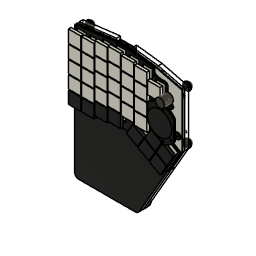
ergothwack-right (requires mirroring) (Autodesk Fusion 360 design; units mm, degrees)
Autodesk Fusion 360 part; units mm, degrees
(part 1 of 6)
sketch "Sketch1" plane through (0, 0, 0) normal (0, 1, 0) x (1, 0, 0)
  line L0 (0, 0) -> (-152.53, 0)
  line L1 (66.3928, -85.1606) -> (66.3928, -83.4672)
  line L2 (66.3928, -83.4672) -> (64.6994, -83.4672)
  line L3 (64.6994, -83.4672) -> (64.6994, -85.1606)
  line L4 (64.6994, -85.1606) -> (66.3928, -85.1606)
  circle A0 centre (65.5461, -86.8539) radius 0.8467
  circle A1 centre (65.5461, -89.3939) radius 0.8467
  circle A2 centre (65.5461, -91.9339) radius 0.8467
  circle A3 centre (65.5461, -94.4739) radius 0.8467
  circle A4 centre (65.5461, -97.0139) radius 0.8467
  circle A5 centre (65.5461, -99.5539) radius 0.8467
  circle A6 centre (65.5461, -102.0939) radius 0.8467
  circle A7 centre (65.5461, -104.6339) radius 0.8467
  circle A8 centre (65.5461, -107.1739) radius 0.8467
  circle A9 centre (65.5461, -109.7139) radius 0.8467
  circle A10 centre (65.5461, -112.2539) radius 0.8467
  line L5 (84.5961, -110.1725) -> (83.3967, -111.3719)
  line L6 (83.3967, -111.3719) -> (84.5961, -112.5714)
  line L7 (84.5961, -112.5714) -> (85.7956, -111.3719)
  line L8 (85.7956, -111.3719) -> (84.5961, -110.1725)
  circle A11 centre (84.5961, -108.8672) radius 0.8467
  circle A12 centre (84.5961, -106.3272) radius 0.8467
  ellipse E0 centre (84.5673, -103.7779) end of major axis (84.5955, -104.6241) minor radius 0.8466
  circle A13 centre (84.5961, -101.2472) radius 0.8467
  circle A14 centre (84.5961, -98.7072) radius 0.8467
  circle A15 centre (84.5961, -96.1672) radius 0.8467
  circle A16 centre (84.5961, -93.6272) radius 0.8467
  circle A17 centre (84.5961, -91.0872) radius 0.8467
  circle A18 centre (84.5961, -88.5472) radius 0.8467
  circle A19 centre (84.5961, -86.0072) radius 0.8467
  circle A20 centre (84.5961, -83.4672) radius 0.8467
  circle A21 centre (83.5378, -112.2539) radius 0.8819
  circle A22 centre (83.5378, -109.7139) radius 0.8819
  circle A23 centre (83.5378, -107.1739) radius 0.8819
  circle A24 centre (83.5378, -104.6339) radius 0.8819
  circle A25 centre (83.5378, -102.0939) radius 0.8819
  circle A26 centre (83.5378, -99.5539) radius 0.8819
  circle A27 centre (83.5378, -97.0139) radius 0.8819
  circle A28 centre (83.5378, -94.4739) radius 0.8819
  circle A29 centre (83.5378, -91.9339) radius 0.8819
  circle A30 centre (83.5378, -89.3939) radius 0.8819
  circle A31 centre (83.5378, -86.8539) radius 0.8819
  circle A32 centre (83.5378, -84.3139) radius 0.8819
  circle A33 centre (68.2978, -84.3139) radius 0.8819
  circle A34 centre (68.2978, -86.8539) radius 0.8819
  circle A35 centre (68.2978, -89.3939) radius 0.8819
  circle A36 centre (68.2978, -91.9339) radius 0.8819
  circle A37 centre (68.2978, -94.4739) radius 0.8819
  circle A38 centre (68.2978, -97.0139) radius 0.8819
  circle A39 centre (68.2978, -99.5539) radius 0.8819
  circle A40 centre (68.2978, -102.0939) radius 0.8819
  circle A41 centre (68.2978, -104.6339) radius 0.8819
  circle A42 centre (68.2978, -107.1739) radius 0.8819
  circle A43 centre (68.2978, -109.7139) radius 0.8819
  circle A44 centre (68.2978, -112.2539) radius 0.8819
  circle A45 centre (80.9978, -89.3939) radius 0.8819
  circle A46 centre (78.4578, -89.3939) radius 0.8819
  circle A47 centre (75.9178, -89.3939) radius 0.8819
  line L9 (86.36, -114.0531) -> (77.3994, -114.0531)
  line L10 (86.36, -81.6328) -> (86.36, -114.0531)
  line L11 (77.3994, -81.6328) -> (86.36, -81.6328)
  line L12 (63.7469, -81.6328) -> (72.7075, -81.6328)
  line L13 (63.7469, -114.0531) -> (63.7469, -81.6681)
  line L14 (72.7075, -114.0531) -> (63.7469, -114.0531)
  circle A48 centre (161.925, -101.6353) radius 0.2469
  circle A49 centre (161.925, -100.8239) radius 0.2469
  circle A50 centre (161.925, -100.0125) radius 0.2469
  circle A51 centre (146.7556, -37.8883) radius 1.5875
  circle A52 centre (115.7464, -33.7256) radius 1.0936
  circle A53 centre (66.4281, -78.105) radius 1.0936
  circle A54 centre (18.8031, -34.0783) radius 1.5875
  circle A55 centre (130.8806, -10.2658) radius 1.5875
  circle A56 centre (123.5781, -102.5878) radius 1.5875
  circle A57 centre (157.6917, -44.4147) radius 1.5875
  circle A58 centre (71.0494, -18.8031) radius 1.0936
  circle A59 centre (95.25, -34.2547) radius 1.0936
  circle A60 centre (146.7556, -76.7997) radius 1.5875
  circle A61 centre (28.3281, -91.2283) radius 1.5875
  circle A62 centre (155.5044, -33.8314) radius 0.8114
  circle A63 centre (155.5044, -36.3714) radius 0.8114
  line L15 (156.3158, -38.5233) -> (156.2806, -38.3822)
  line L16 (156.2806, -38.3822) -> (156.21, -38.2764)
  line L17 (156.21, -38.2764) -> (156.1042, -38.1706)
  line L18 (156.1042, -38.1706) -> (155.9983, -38.1)
  line L19 (155.9983, -38.1) -> (155.8572, -38.0647)
  line L20 (155.8572, -38.0647) -> (155.0458, -38.0647)
  line L21 (155.0458, -38.0647) -> (154.9047, -38.1)
  line L22 (154.9047, -38.1) -> (154.7989, -38.1706)
  line L23 (154.7989, -38.1706) -> (154.6931, -38.2764)
  line L24 (154.6931, -38.2764) -> (154.6225, -38.3822)
  line L25 (154.6225, -38.3822) -> (154.5872, -38.5233)
  line L26 (154.5872, -38.5233) -> (154.5872, -39.3347)
  line L27 (154.5872, -39.3347) -> (154.6225, -39.4758)
  line L28 (154.6225, -39.4758) -> (154.6931, -39.5817)
  line L29 (154.6931, -39.5817) -> (154.7989, -39.6875)
  line L30 (154.7989, -39.6875) -> (154.9047, -39.7581)
  line L31 (154.9047, -39.7581) -> (155.0458, -39.7933)
  line L32 (155.0458, -39.7933) -> (155.8572, -39.7933)
  line L33 (155.8572, -39.7933) -> (155.9983, -39.7581)
  line L34 (155.9983, -39.7581) -> (156.1042, -39.6875)
  line L35 (156.1042, -39.6875) -> (156.21, -39.5817)
  line L36 (156.21, -39.5817) -> (156.2806, -39.4758)
  line L37 (156.2806, -39.4758) -> (156.3158, -39.3347)
  line L38 (156.3158, -39.3347) -> (156.3158, -38.5233)
  circle A64 centre (84.5961, -83.4672) radius 0.8467
  circle A65 centre (84.5961, -86.0072) radius 0.8467
  circle A66 centre (84.5961, -88.5472) radius 0.8467
  circle A67 centre (84.5961, -91.0872) radius 0.8467
  circle A68 centre (84.5961, -93.6272) radius 0.8467
  circle A69 centre (84.5961, -96.1672) radius 0.8467
  circle A70 centre (84.5961, -98.7072) radius 0.8467
  circle A71 centre (84.5961, -101.2472) radius 0.8467
  circle A72 centre (84.5961, -103.7872) radius 0.8467
  circle A73 centre (84.5961, -106.3272) radius 0.8467
  circle A74 centre (84.5961, -108.8672) radius 0.8467
  line L39 (85.4428, -112.2539) -> (85.4428, -110.5253)
  line L40 (85.4428, -110.5253) -> (83.7494, -110.5253)
  line L41 (83.7494, -110.5253) -> (83.7494, -112.2186)
  line L42 (83.7494, -112.2186) -> (85.4428, -112.2186)
  line L43 (85.4428, -112.2186) -> (85.4428, -112.2539)
  circle A75 centre (65.5461, -112.2539) radius 0.8467
  circle A76 centre (65.5461, -109.7139) radius 0.8467
  circle A77 centre (65.5461, -107.1739) radius 0.8467
  circle A78 centre (65.5461, -104.6339) radius 0.8467
  circle A79 centre (65.5461, -102.0939) radius 0.8467
  circle A80 centre (65.5461, -99.5539) radius 0.8467
  circle A81 centre (65.5461, -97.0139) radius 0.8467
  circle A82 centre (65.5461, -94.4739) radius 0.8467
  circle A83 centre (65.5461, -91.9339) radius 0.8467
  circle A84 centre (65.5461, -89.3939) radius 0.8467
  circle A85 centre (65.5461, -86.8539) radius 0.8467
  line L44 (64.6994, -83.4672) -> (64.6994, -85.1606)
  line L45 (64.6994, -85.1606) -> (66.3928, -85.1606)
  line L46 (66.3928, -85.1606) -> (66.3928, -83.4672)
  line L47 (66.3928, -83.4672) -> (64.6994, -83.4672)
  line L48 (130.5278, -107.2444) -> (130.3161, -106.5036)
  line L49 (125.6947, -108.5497) -> (125.483, -107.8089)
  line L50 (160.3728, -84.2433) -> (160.3728, -83.5025)
  line L51 (155.3633, -84.2433) -> (155.3633, -83.5025)
  line L52 (160.3728, -77.7169) -> (160.3728, -76.9761)
  line L53 (155.3633, -77.7169) -> (155.3633, -76.9761)
  circle A86 centre (148.6606, -21.9781) radius 2.6106
  circle A87 centre (139.1356, -5.4681) radius 2.6106
  circle A88 centre (114.3353, -19.7908) radius 2.6106
  circle A89 centre (83.5731, -29.3158) radius 2.6106
  circle A90 centre (56.9031, -29.3158) radius 2.6106
  circle A91 centre (37.8531, -24.5533) radius 2.6106
  circle A92 centre (18.8031, -24.5533) radius 2.6106
  circle A93 centre (132.1506, -31.5383) radius 2.6106
  circle A94 centre (114.0531, -45.9669) radius 2.6106
  circle A95 centre (95.0031, -48.3658) radius 2.6106
  circle A96 centre (75.9531, -50.7294) radius 2.6106
  circle A97 centre (56.9031, -48.3658) radius 2.6106
  circle A98 centre (37.8531, -43.6033) radius 2.6106
  circle A99 centre (18.8031, -43.6033) radius 2.6106
  circle A100 centre (133.1031, -55.4919) radius 2.6106
  circle A101 centre (114.0531, -65.0169) radius 2.6106
  circle A102 centre (95.0031, -67.4158) radius 2.6106
  circle A103 centre (75.9531, -69.7794) radius 2.6106
  circle A104 centre (56.9031, -67.4158) radius 2.6106
  circle A105 centre (37.8531, -62.6533) radius 2.6106
  circle A106 centre (18.8031, -62.6533) radius 2.6106
  circle A107 centre (133.1031, -74.5419) radius 2.6106
  circle A108 centre (114.0531, -84.0669) radius 2.6106
  circle A109 centre (95.0031, -86.4658) radius 2.6106
  circle A110 centre (75.9531, -88.8294) radius 2.6106
  circle A111 centre (56.9031, -86.4658) radius 2.6106
  circle A112 centre (37.8531, -81.7033) radius 2.6106
  circle A113 centre (18.8031, -81.7033) radius 2.6106
  circle A114 centre (133.1031, -93.5919) radius 2.6106
  circle A115 centre (114.0531, -103.1169) radius 2.6106
  circle A116 centre (95.0031, -105.5158) radius 2.6106
  circle A117 centre (75.9531, -107.8794) radius 2.6106
  circle A118 centre (56.9031, -105.5158) radius 2.6106
  circle A119 centre (37.8531, -100.7533) radius 2.6106
  circle A120 centre (18.8031, -100.7533) radius 2.6106
  circle A121 centre (155.5044, -66.5339) radius 0.8114
  circle A122 centre (155.5044, -69.0739) radius 0.8114
  line L54 (156.3158, -71.1906) -> (156.2806, -71.0494)
  line L55 (156.2806, -71.0494) -> (156.21, -70.9436)
  line L56 (156.21, -70.9436) -> (156.1042, -70.8378)
  line L57 (156.1042, -70.8378) -> (155.9983, -70.7672)
  line L58 (155.9983, -70.7672) -> (155.8572, -70.7319)
  line L59 (155.8572, -70.7319) -> (155.0458, -70.7319)
  line L60 (155.0458, -70.7319) -> (154.9047, -70.7672)
  line L61 (154.9047, -70.7672) -> (154.7989, -70.8378)
  line L62 (154.7989, -70.8378) -> (154.6931, -70.9436)
  line L63 (154.6931, -70.9436) -> (154.6225, -71.0494)
  line L64 (154.6225, -71.0494) -> (154.5872, -71.1906)
  line L65 (154.5872, -71.1906) -> (154.5872, -72.0019)
  line L66 (154.5872, -72.0019) -> (154.6225, -72.1431)
  line L67 (154.6225, -72.1431) -> (154.6931, -72.2489)
  line L68 (154.6931, -72.2489) -> (154.7989, -72.3547)
  line L69 (154.7989, -72.3547) -> (154.9047, -72.4253)
  line L70 (154.9047, -72.4253) -> (155.0458, -72.4606)
  line L71 (155.0458, -72.4606) -> (155.8572, -72.4606)
  line L72 (155.8572, -72.4606) -> (155.9983, -72.4253)
  line L73 (155.9983, -72.4253) -> (156.1042, -72.3547)
  line L74 (156.1042, -72.3547) -> (156.21, -72.2489)
  line L75 (156.21, -72.2489) -> (156.2806, -72.1431)
  line L76 (156.2806, -72.1431) -> (156.3158, -72.0019)
  line L77 (156.3158, -72.0019) -> (156.3158, -71.1906)
  circle A123 centre (159.2086, -57.9967) radius 0.9878
  circle A124 centre (159.2086, -52.9872) radius 0.9878
  line L78 (150.6008, -60.0781) -> (150.6008, -62.0889)
  line L79 (150.6008, -62.0889) -> (153.8111, -62.0889)
  line L80 (153.8111, -62.0889) -> (153.8111, -60.0781)
  line L81 (153.8111, -60.0781) -> (150.6008, -60.0781)
  line L82 (150.6008, -48.895) -> (150.6008, -50.9058)
  line L83 (150.6008, -50.9058) -> (153.8111, -50.9058)
  line L84 (153.8111, -50.9058) -> (153.8111, -48.895)
  line L85 (153.8111, -48.895) -> (150.6008, -48.895)
  circle A125 centre (144.7094, -55.4919) radius 0.9878
  circle A126 centre (144.7094, -52.9872) radius 0.9878
  line L86 (143.6864, -57.0089) -> (143.6864, -59.0197)
  line L87 (143.6864, -59.0197) -> (145.6972, -59.0197)
  line L88 (145.6972, -59.0197) -> (145.6972, -57.0089)
  line L89 (145.6972, -57.0089) -> (143.6864, -57.0089)
  circle A127 centre (159.2086, -96.0967) radius 0.9878
  circle A128 centre (159.2086, -91.0872) radius 0.9878
  line L90 (150.6008, -98.1781) -> (150.6008, -100.1889)
  line L91 (150.6008, -100.1889) -> (153.8111, -100.1889)
  line L92 (153.8111, -100.1889) -> (153.8111, -98.1781)
  line L93 (153.8111, -98.1781) -> (150.6008, -98.1781)
  line L94 (150.6008, -86.995) -> (150.6008, -89.0058)
  line L95 (150.6008, -89.0058) -> (153.8111, -89.0058)
  line L96 (153.8111, -89.0058) -> (153.8111, -86.995)
  line L97 (153.8111, -86.995) -> (150.6008, -86.995)
  circle A129 centre (144.7094, -93.5919) radius 0.9878
  circle A130 centre (144.7094, -91.0872) radius 0.9878
  line L98 (143.6864, -95.1089) -> (143.6864, -97.1197)
  line L99 (143.6864, -97.1197) -> (145.6972, -97.1197)
  line L100 (145.6972, -97.1197) -> (145.6972, -95.1089)
  line L101 (145.6972, -95.1089) -> (143.6864, -95.1089)
  circle A131 centre (104.4928, -83.82) radius 0.8467
  line L102 (105.3394, -87.2067) -> (105.3394, -85.5133)
  line L103 (105.3394, -85.5133) -> (103.6461, -85.5133)
  line L104 (103.6461, -85.5133) -> (103.6461, -87.2067)
  line L105 (103.6461, -87.2067) -> (105.3394, -87.2067)
  line L106 (81.4211, -132.3975) -> (92.2514, -132.3975)
  line L107 (92.2514, -132.3975) -> (92.2514, -130.81)
  line L108 (92.2514, -130.81) -> (81.4211, -130.81)
  line L109 (81.4211, -130.81) -> (81.4211, -132.3975)
  line L110 (81.1389, -132.6092) -> (92.5336, -132.6092)
  line L111 (92.5336, -132.6092) -> (92.5336, -130.5983)
  line L112 (92.5336, -130.5983) -> (81.1389, -130.5983)
  line L113 (81.1389, -130.5983) -> (81.1389, -132.6092)
  line L114 (161.7839, -117.9336) -> (161.7839, -131.1628)
  line L115 (9.2428, -117.9336) -> (9.2428, -131.1628)
  line L116 (161.7839, -117.9336) -> (161.7839, -121.92)
  line L117 (9.2428, -117.9336) -> (9.2428, -123.5781)
  line L118 (81.4211, -131.5861) -> (92.2514, -131.5861)
  line L119 (92.2514, -131.5861) -> (92.2514, -129.9986)
  line L120 (92.2514, -129.9986) -> (81.4211, -129.9986)
  line L121 (81.4211, -129.9986) -> (81.4211, -131.5861)
  line L122 (81.1389, -131.7978) -> (92.5336, -131.7978)
  line L123 (92.5336, -131.7978) -> (92.5336, -129.7869)
  line L124 (92.5336, -129.7869) -> (81.1389, -129.7869)
  line L125 (81.1389, -129.7869) -> (81.1389, -131.7978)
  line L126 (80.9978, -130.4925) -> (80.4333, -130.4925)
  line L127 (80.6803, -130.4925) -> (80.6803, -131.4803)
  line L128 (80.6803, -131.4803) -> (80.5744, -131.3392)
  line L129 (80.6097, -131.3392) -> (80.5039, -131.2333)
  line L130 (80.5039, -131.2333) -> (80.3981, -131.1981)
  line L131 (81.8797, -131.4803) -> (81.4211, -131.4803)
  line L132 (81.4211, -131.4803) -> (81.3858, -131.0217)
  line L133 (81.3506, -130.9864) -> (81.3858, -131.0217)
  line L134 (81.4211, -131.0569) -> (81.5269, -131.0922)
  line L135 (81.4917, -131.0922) -> (81.7386, -131.0922)
  line L136 (81.7386, -131.0922) -> (81.8444, -131.0569)
  line L137 (81.8444, -131.0569) -> (81.8797, -131.0217)
  line L138 (81.8797, -130.9864) -> (81.915, -130.8806)
  line L139 (81.9503, -130.9158) -> (81.9503, -130.6689)
  line L140 (81.9503, -130.6689) -> (81.915, -130.5631)
  line L141 (81.8797, -130.5631) -> (81.8444, -130.5278)
  line L142 (81.8444, -130.5278) -> (81.7386, -130.4925)
  line L143 (81.7386, -130.4925) -> (81.4917, -130.4925)
  line L144 (81.4917, -130.4925) -> (81.3858, -130.5278)
  line L145 (81.4211, -130.5278) -> (81.3858, -130.5631)
  line L146 (82.3031, -131.3744) -> (82.3383, -131.4097)
  line L147 (82.3736, -131.445) -> (82.4794, -131.4803)
  line L148 (82.4442, -131.4803) -> (82.6911, -131.4803)
  line L149 (82.6911, -131.4803) -> (82.7969, -131.445)
  line L150 (82.7969, -131.445) -> (82.8322, -131.4097)
  line L151 (82.8322, -131.3744) -> (82.8675, -131.2686)
  line L152 (82.9028, -131.3039) -> (82.9028, -131.1981)
  line L153 (82.9028, -131.1981) -> (82.8675, -131.0569)
  line L154 (82.8322, -131.0569) -> (82.2678, -130.4925)
  line L155 (82.2678, -130.4925) -> (82.9028, -130.4925)
  line L156 (83.3261, -130.5631) -> (83.3614, -130.5278)
  line L157 (83.3614, -130.5278) -> (83.3261, -130.4925)
  line L158 (83.3261, -130.4925) -> (83.2908, -130.5278)
  line L159 (83.2556, -130.5278) -> (83.2908, -130.5631)
  line L160 (83.3261, -130.5631) -> (83.3261, -130.4572)
  line L161 (84.2786, -131.4803) -> (83.82, -131.4803)
  line L162 (83.7847, -131.4803) -> (83.7494, -131.0217)
  line L163 (83.7494, -130.9864) -> (83.7847, -131.0217)
  line L164 (83.7847, -131.0569) -> (83.8906, -131.0922)
  line L165 (83.8906, -131.0922) -> (84.1375, -131.0922)
  line L166 (84.1375, -131.0922) -> (84.2433, -131.0569)
  line L167 (84.2081, -131.0569) -> (84.2433, -131.0217)
  line L168 (84.2786, -130.9864) -> (84.3139, -130.8806)
  line L169 (84.3139, -130.9158) -> (84.3139, -130.6689)
  line L170 (84.3139, -130.6689) -> (84.2786, -130.5631)
  line L171 (84.2786, -130.5631) -> (84.2433, -130.5278)
  line L172 (84.2081, -130.5278) -> (84.1022, -130.4925)
  line L173 (84.1375, -130.4925) -> (83.8906, -130.4925)
  line L174 (83.8906, -130.4925) -> (83.7847, -130.5278)
  line L175 (83.7847, -130.5278) -> (83.7494, -130.5631)
  line L176 (84.6314, -131.4803) -> (85.2664, -131.4803)
  line L177 (85.2664, -131.4803) -> (84.9489, -131.0922)
  line L178 (84.9489, -131.0922) -> (85.09, -131.0922)
  line L179 (85.09, -131.0922) -> (85.1958, -131.0569)
  line L180 (85.1606, -131.0569) -> (85.1958, -131.0217)
  line L181 (85.2311, -130.9864) -> (85.2664, -130.8806)
  line L182 (85.2664, -130.9158) -> (85.2664, -130.6689)
  line L183 (85.2664, -130.6689) -> (85.2311, -130.5631)
  line L184 (85.2311, -130.5631) -> (85.1958, -130.5278)
  line L185 (85.1606, -130.5278) -> (85.0547, -130.4925)
  line L186 (85.09, -130.4925) -> (84.8078, -130.4925)
  line L187 (84.8078, -130.4925) -> (84.7019, -130.5278)
  line L188 (84.7019, -130.5278) -> (84.6667, -130.5631)
  line L189 (85.9014, -131.4803) -> (86.0072, -131.4803)
  line L190 (85.9719, -131.4803) -> (86.0778, -131.445)
  line L191 (86.0778, -131.445) -> (86.1131, -131.4097)
  line L192 (86.1131, -131.3744) -> (86.1483, -131.2686)
  line L193 (86.1836, -131.3039) -> (86.2189, -131.1275)
  line L194 (86.2189, -131.0922) -> (86.2189, -130.8453)
  line L195 (86.2189, -130.8453) -> (86.1836, -130.6689)
  line L196 (86.1836, -130.6689) -> (86.1483, -130.5631)
  line L197 (86.1131, -130.5631) -> (86.0778, -130.5278)
  line L198 (86.0778, -130.5278) -> (85.9719, -130.4925)
  line L199 (85.9719, -130.4925) -> (85.8661, -130.4925)
  line L200 (85.9014, -130.4925) -> (85.7956, -130.5278)
  line L201 (85.7956, -130.5278) -> (85.7603, -130.5631)
  line L202 (85.7603, -130.5631) -> (85.725, -130.6689)
  line L203 (85.6897, -130.6689) -> (85.6544, -130.8453)
  line L204 (85.6544, -130.8453) -> (85.6544, -131.0922)
  line L205 (85.6544, -131.0922) -> (85.6897, -131.2686)
  line L206 (85.6897, -131.3039) -> (85.725, -131.4097)
  line L207 (85.7603, -131.3744) -> (85.7956, -131.4097)
  line L208 (85.7956, -131.445) -> (85.9014, -131.4803)
  line L209 (86.8539, -131.4803) -> (86.9597, -131.4803)
  line L210 (86.9244, -131.4803) -> (87.0303, -131.445)
  line L211 (87.0303, -131.445) -> (87.0656, -131.4097)
  line L212 (87.0656, -131.3744) -> (87.1008, -131.2686)
  line L213 (87.1361, -131.3039) -> (87.1714, -131.1275)
  line L214 (87.1714, -131.0922) -> (87.1714, -130.8453)
  line L215 (87.1714, -130.8453) -> (87.1361, -130.6689)
  line L216 (87.1361, -130.6689) -> (87.1008, -130.5631)
  line L217 (87.0656, -130.5631) -> (87.0303, -130.5278)
  line L218 (87.0303, -130.5278) -> (86.9244, -130.4925)
  line L219 (86.9244, -130.4925) -> (86.8186, -130.4925)
  line L220 (86.8539, -130.4925) -> (86.7481, -130.5278)
  line L221 (86.7481, -130.5278) -> (86.7128, -130.5631)
  line L222 (86.7128, -130.5631) -> (86.6775, -130.6689)
  line L223 (86.6422, -130.6689) -> (86.6069, -130.8453)
  line L224 (86.6069, -130.8453) -> (86.6069, -131.0922)
  line L225 (86.6069, -131.0922) -> (86.6422, -131.2686)
  line L226 (86.6422, -131.3039) -> (86.6775, -131.4097)
  line L227 (86.7128, -131.3744) -> (86.7481, -131.4097)
  line L228 (86.7481, -131.445) -> (86.8539, -131.4803)
  line L229 (88.3708, -130.4925) -> (88.3708, -131.1628)
  line L230 (88.3708, -131.0569) -> (88.4061, -131.0922)
  line L231 (88.4061, -131.0922) -> (88.5119, -131.1275)
  line L232 (88.5119, -131.1275) -> (88.6531, -131.1275)
  line L233 (88.6531, -131.1275) -> (88.7589, -131.0922)
  line L234 (88.7589, -131.0922) -> (88.7942, -130.9864)
  line L235 (88.7942, -130.9864) -> (88.7942, -130.4572)
  line L236 (88.7942, -130.9864) -> (88.8294, -131.0922)
  line L237 (88.8294, -131.0922) -> (88.9353, -131.1275)
  line L238 (88.9353, -131.1275) -> (89.0764, -131.1275)
  line L239 (89.0764, -131.1275) -> (89.1822, -131.0922)
  line L240 (89.1822, -131.0922) -> (89.2175, -130.9864)
  line L241 (89.2175, -130.9864) -> (89.2175, -130.4572)
  line L242 (89.7114, -130.4925) -> (89.7114, -131.1628)
  line L243 (89.7114, -131.0569) -> (89.7467, -131.0922)
  line L244 (89.7467, -131.0922) -> (89.8525, -131.1275)
  line L245 (89.8525, -131.1275) -> (89.9936, -131.1275)
  line L246 (89.9936, -131.1275) -> (90.0994, -131.0922)
  line L247 (90.0642, -131.0922) -> (90.0994, -130.9864)
  line L248 (90.1347, -130.9864) -> (90.1347, -130.4572)
  line L249 (90.1347, -130.9864) -> (90.17, -131.0922)
  line L250 (90.17, -131.0922) -> (90.2758, -131.1275)
  line L251 (90.2758, -131.1275) -> (90.4169, -131.1275)
  line L252 (90.4169, -131.1275) -> (90.5228, -131.0922)
  line L253 (90.4875, -131.0922) -> (90.5228, -130.9864)
  line L254 (90.5581, -130.9864) -> (90.5581, -130.4572)
  line L255 (9.2428, -110.8075) -> (9.2428, -130.3514)
  line L256 (161.7839, -110.8075) -> (161.7839, -130.3514)
  line L257 (9.2428, -129.7869) -> (161.7839, -129.7869)
  line L258 (9.2428, -129.7869) -> (161.7839, -129.7869)
  line L259 (9.2428, -129.7869) -> (10.3717, -130.3867)
  line L260 (9.2428, -129.7869) -> (10.3717, -129.1872)
  line L261 (161.7839, -129.7869) -> (160.655, -129.1872)
  line L262 (161.7839, -129.7869) -> (160.655, -130.3867)
  line L263 (161.7839, -103.1522) -> (161.7839, -110.3136)
  line L264 (-3.474, -61.5853) -> (-3.474, -63.702)
  line L265 (-3.474, -63.702) -> (3.9344, -63.702)
  line L266 (3.9344, -63.702) -> (3.9344, -61.5853)
  line L267 (3.9344, -61.5853) -> (-3.474, -61.5853)
  line L268 (-3.6856, -61.3031) -> (-3.6856, -63.9842)
  line L269 (-3.6856, -63.9842) -> (4.146, -63.9842)
  line L270 (4.146, -63.9842) -> (4.146, -61.3031)
  line L271 (4.146, -61.3031) -> (-3.6856, -61.3031)
  line L272 (0.635, -58.1378) -> (0.635, -58.3142)
  line L273 (0.635, -58.3142) -> (0.5997, -58.42)
  line L274 (0.5997, -58.42) -> (0.5644, -58.4553)
  line L275 (0.5644, -58.4553) -> (0.4233, -58.5611)
  line L276 (0.4233, -58.5611) -> (0.2469, -58.5964)
  line L277 (0.2117, -58.5964) -> (-0.1764, -58.5964)
  line L278 (-0.1764, -58.5964) -> (-0.2822, -58.5611)
  line L279 (-0.2469, -58.5611) -> (-0.2822, -58.5258)
  line L280 (-0.3175, -58.5258) -> (-0.3528, -58.42)
  line L281 (-0.3528, -58.42) -> (-0.3528, -58.2436)
  line L282 (-0.3528, -58.2083) -> (-0.3175, -58.1025)
  line L283 (-0.3175, -58.1378) -> (-0.2822, -58.1025)
  line L284 (-0.2469, -58.0672) -> (-0.1411, -58.0319)
  line L285 (-0.1764, -58.0319) -> (0.0706, -58.0319)
  line L286 (0.0706, -58.0319) -> (0.1764, -58.0672)
  line L287 (0.1764, -58.0672) -> (0.2117, -58.1025)
  line L288 (0.2117, -58.1378) -> (0.2469, -58.2436)
  line L289 (0.2469, -58.2083) -> (0.2469, -58.3847)
  line L290 (0.2469, -58.42) -> (0.2117, -58.5258)
  line L291 (0.2117, -58.5258) -> (0.1764, -58.5611)
  line L292 (0.1764, -58.5611) -> (0.0706, -58.5964)
  line L293 (-0.3528, -59.5136) -> (-0.3528, -59.055)
  line L294 (-0.3528, -59.0197) -> (0.1058, -58.9844)
  line L295 (0.1058, -58.9844) -> (0.0706, -59.0197)
  line L296 (0.0706, -59.0197) -> (0.0353, -59.1256)
  line L297 (0.0353, -59.1256) -> (0.0353, -59.3725)
  line L298 (0.0353, -59.3725) -> (0.0706, -59.4783)
  line L299 (0.0706, -59.4783) -> (0.1058, -59.5136)
  line L300 (0.1058, -59.5136) -> (0.2117, -59.5489)
  line L301 (0.2117, -59.5489) -> (0.4586, -59.5489)
  line L302 (0.4586, -59.5489) -> (0.5644, -59.5136)
  line L303 (0.5644, -59.5136) -> (0.5997, -59.4783)
  line L304 (0.5997, -59.4783) -> (0.635, -59.3725)
  line L305 (0.635, -59.3725) -> (0.635, -59.1256)
  line L306 (0.635, -59.1256) -> (0.5997, -59.0197)
  line L307 (0.5997, -59.0197) -> (0.5644, -58.9844)
  line L308 (0.5644, -59.9722) -> (0.5997, -60.0075)
  line L309 (0.5997, -60.0428) -> (0.635, -60.0075)
  line L310 (0.635, -59.9722) -> (0.5997, -59.9369)
  line L311 (0.5997, -59.9369) -> (0.5644, -59.9722)
  line L312 (0.5644, -59.9722) -> (0.6703, -59.9722)
  line L313 (-0.3528, -60.3603) -> (-0.3528, -60.9953)
  line L314 (-0.3528, -60.9953) -> (0.0353, -60.6778)
  line L315 (0.0353, -60.6425) -> (0.0353, -60.7836)
  line L316 (0.0353, -60.7836) -> (0.0706, -60.8894)
  line L317 (0.0706, -60.8894) -> (0.1058, -60.9247)
  line L318 (0.1058, -60.9247) -> (0.2117, -60.96)
  line L319 (0.2117, -60.9953) -> (0.4586, -60.9953)
  line L320 (0.4586, -60.9953) -> (0.5644, -60.96)
  line L321 (0.5644, -60.9247) -> (0.5997, -60.8894)
  line L322 (0.5997, -60.8894) -> (0.635, -60.7836)
  line L323 (0.635, -60.7836) -> (0.635, -60.5014)
  line L324 (0.635, -60.5014) -> (0.5997, -60.4308)
  line L325 (0.5997, -60.4308) -> (0.5644, -60.3956)
  line L326 (-0.0353, -61.8419) -> (0.635, -61.8419)
  line L327 (-0.3881, -61.595) -> (0.3175, -61.3481)
  line L328 (0.3175, -61.3833) -> (0.3175, -62.0183)
  line L329 (-0.3528, -62.5475) -> (-0.3528, -62.6533)
  line L330 (-0.3528, -62.6533) -> (-0.3175, -62.7592)
  line L331 (-0.3175, -62.7592) -> (-0.2822, -62.7944)
  line L332 (-0.2469, -62.7944) -> (-0.1411, -62.8297)
  line L333 (-0.1764, -62.8297) -> (0, -62.865)
  line L334 (0.0353, -62.9003) -> (0.2822, -62.9003)
  line L335 (0.2469, -62.9003) -> (0.4233, -62.865)
  line L336 (0.4586, -62.8297) -> (0.5644, -62.7944)
  line L337 (0.5644, -62.7944) -> (0.5997, -62.7592)
  line L338 (0.5997, -62.7592) -> (0.635, -62.6533)
  line L339 (0.635, -62.6533) -> (0.635, -62.5475)
  line L340 (0.635, -62.5475) -> (0.5997, -62.4417)
  line L341 (0.5997, -62.4769) -> (0.5644, -62.4417)
  line L342 (0.5644, -62.4064) -> (0.4586, -62.3711)
  line L343 (0.4586, -62.3711) -> (0.2822, -62.3358)
  line L344 (0.2469, -62.3358) -> (0.0353, -62.3358)
  line L345 (0.0353, -62.3358) -> (-0.1411, -62.3711)
  line L346 (-0.1764, -62.3711) -> (-0.2822, -62.4064)
  line L347 (-0.2469, -62.4064) -> (-0.2822, -62.4417)
  line L348 (-0.3175, -62.4769) -> (-0.3528, -62.5475)
  line L349 (-0.3528, -63.5) -> (-0.3528, -63.6058)
  line L350 (-0.3528, -63.6058) -> (-0.3175, -63.7117)
  line L351 (-0.3175, -63.7117) -> (-0.2822, -63.7469)
  line L352 (-0.2469, -63.7469) -> (-0.1411, -63.7822)
  line L353 (-0.1764, -63.7822) -> (0, -63.8175)
  line L354 (0.0353, -63.8528) -> (0.2822, -63.8528)
  line L355 (0.2469, -63.8528) -> (0.4233, -63.8175)
  line L356 (0.4586, -63.7822) -> (0.5644, -63.7469)
  line L357 (0.5644, -63.7469) -> (0.5997, -63.7117)
  line L358 (0.5997, -63.7117) -> (0.635, -63.6058)
  line L359 (0.635, -63.6058) -> (0.635, -63.5)
  line L360 (0.635, -63.5) -> (0.5997, -63.3942)
  line L361 (0.5997, -63.4294) -> (0.5644, -63.3942)
  line L362 (0.5644, -63.3589) -> (0.4586, -63.3236)
  line L363 (0.4586, -63.3236) -> (0.2822, -63.2883)
  line L364 (0.2469, -63.2883) -> (0.0353, -63.2883)
  line L365 (0.0353, -63.2883) -> (-0.1411, -63.3236)
  line L366 (-0.1764, -63.3236) -> (-0.2822, -63.3589)
  line L367 (-0.2469, -63.3589) -> (-0.2822, -63.3942)
  line L368 (-0.3175, -63.4294) -> (-0.3528, -63.5353)
  line L369 (0.635, -65.0169) -> (-0.0353, -65.0169)
  line L370 (0.0706, -65.0169) -> (0.0353, -65.0522)
  line L371 (0.0353, -65.0875) -> (0, -65.1933)
  line L372 (-0.0353, -65.1581) -> (-0.0353, -65.2992)
  line L373 (-0.0353, -65.3344) -> (0, -65.4403)
  line L374 (0.0353, -65.405) -> (0.1411, -65.4403)
  line L375 (0.1058, -65.4756) -> (0.635, -65.4756)
  line L376 (0.1058, -65.4756) -> (0, -65.5108)
  line L377 (0.0353, -65.5108) -> (0, -65.6167)
  line L378 (-0.0353, -65.6167) -> (-0.0353, -65.7578)
  line L379 (-0.0353, -65.7578) -> (0, -65.8636)
  line L380 (0.0353, -65.8283) -> (0.1411, -65.8636)
  line L381 (0.1058, -65.8989) -> (0.635, -65.8989)
  line L382 (0.635, -66.3575) -> (-0.0353, -66.3575)
  line L383 (0.0706, -66.3575) -> (0.0353, -66.4281)
  line L384 (0.0353, -66.4281) -> (0, -66.5339)
  line L385 (-0.0353, -66.4986) -> (-0.0353, -66.6397)
  line L386 (-0.0353, -66.6397) -> (0, -66.7456)
  line L387 (0.0353, -66.7456) -> (0.1411, -66.7808)
  line L388 (0.1058, -66.7808) -> (0.635, -66.7808)
  line L389 (0.1058, -66.7808) -> (0, -66.8161)
  line L390 (0.0353, -66.8514) -> (0, -66.9572)
  line L391 (-0.0353, -66.9219) -> (-0.0353, -67.063)
  line L392 (-0.0353, -67.063) -> (0, -67.1689)
  line L393 (0.0353, -67.1689) -> (0.1411, -67.2042)
  line L394 (0.1058, -67.2394) -> (0.635, -67.2394)
  line L395 (8.7489, -14.9931) -> (0.7408, -14.9931)
  line L396 (8.7489, -110.3136) -> (0.7408, -110.3136)
  line L397 (1.3406, -14.9931) -> (1.3406, -110.3136)
  line L398 (1.3406, -14.9931) -> (1.3406, -110.3136)
  line L399 (1.3406, -14.9931) -> (0.7408, -16.122)
  line L400 (1.3406, -14.9931) -> (1.9403, -16.122)
  line L401 (1.3406, -110.3136) -> (1.9403, -109.1847)
  line L402 (1.3406, -110.3136) -> (0.7408, -109.1847)
  circle A132 centre (66.4281, -78.105) radius 0.9878
  circle A133 centre (115.7464, -33.7256) radius 0.9878
  circle A134 centre (95.25, -34.2547) radius 0.9878
  circle A135 centre (71.0494, -18.8031) radius 0.9878
  circle A136 centre (28.3281, -91.2283) radius 1.5169
  circle A137 centre (18.8031, -34.0783) radius 1.5169
  circle A138 centre (130.9158, -10.2658) radius 1.5169
  circle A139 centre (146.7556, -76.7997) radius 1.5169
  circle A140 centre (157.6917, -44.4147) radius 1.5169
  circle A141 centre (146.7556, -37.8883) radius 1.5169
  circle A142 centre (123.5781, -102.5878) radius 1.5169
  line L403 (9.2428, -105.6569) -> (9.2428, -19.6497)
  line L404 (161.7839, -30.1978) -> (161.7839, -98.4956)
  line L405 (77.8933, -14.9931) -> (103.8578, -14.9931)
  line L406 (9.2428, -14.9931) -> (73.2367, -14.9931)
  line L407 (66.9572, -117.4397) -> (9.2428, -110.3136)
  line L408 (84.9842, -117.4397) -> (66.9572, -117.4397)
  line L409 (123.6133, -112.6772) -> (84.9842, -117.4397)
  line L410 (161.7839, -103.1522) -> (123.6486, -112.6772)
  line L411 (142.6281, 7.5847) -> (103.8578, -14.9931)
  line L412 (161.7839, -25.5411) -> (142.6281, 7.62)
  line L413 (81.4286, 6.2604) -> (95.5897, 6.2604) construction
  line L414 (95.5897, 6.2604) -> (95.5897, 9.7882) construction
  line L415 (95.5897, 9.7882) -> (81.4286, 9.7882) construction
  line L416 (81.4286, 9.7882) -> (81.4286, 6.2604) construction
  line L417 (87.0025, 6.2604) -> (87.0042, 6.2604) construction
  line L418 (87.0042, 6.2604) -> (87.0042, 9.7882) construction
  line L419 (87.0042, 9.7882) -> (87.0025, 9.7882) construction
  line L420 (87.0025, 9.7882) -> (87.0025, 6.2604) construction
  line L421 (90.0364, 6.2604) -> (95.4538, 6.2604) construction
  line L422 (95.4538, 6.2604) -> (95.4538, 9.7882) construction
  line L423 (95.4538, 9.7882) -> (90.0364, 9.7882) construction
  line L424 (90.0364, 9.7882) -> (90.0364, 6.2604) construction
  line L425 (81.1468, 6.4733) -> (95.3079, 6.4733) construction
  line L426 (95.3079, 6.4733) -> (95.3079, 10.0011) construction
  line L427 (95.3079, 10.0011) -> (81.1468, 10.0011) construction
  line L428 (81.1468, 10.0011) -> (81.1468, 6.4733) construction
  line L429 (86.7207, 6.4733) -> (86.7224, 6.4733) construction
  line L430 (86.7224, 6.4733) -> (86.7224, 10.0011) construction
  line L431 (86.7224, 10.0011) -> (86.7207, 10.0011) construction
  line L432 (86.7207, 10.0011) -> (86.7207, 6.4733) construction
  line L433 (90.319, 6.4733) -> (95.7365, 6.4733) construction
  line L434 (95.7365, 6.4733) -> (95.7365, 10.0011) construction
  line L435 (95.7365, 10.0011) -> (90.319, 10.0011) construction
  line L436 (90.319, 10.0011) -> (90.319, 6.4733) construction
  line L437 (81.4286, 5.4429) -> (95.5897, 5.4429) construction
  line L438 (95.5897, 5.4429) -> (95.5897, 8.9706) construction
  line L439 (95.5897, 8.9706) -> (81.4286, 8.9706) construction
  line L440 (81.4286, 8.9706) -> (81.4286, 5.4429) construction
  line L441 (87.0025, 5.4429) -> (87.0042, 5.4429) construction
  line L442 (87.0042, 5.4429) -> (87.0042, 8.9706) construction
  line L443 (87.0042, 8.9706) -> (87.0025, 8.9706) construction
  line L444 (87.0025, 8.9706) -> (87.0025, 5.4429) construction
  line L445 (90.0364, 5.4429) -> (95.4538, 5.4429) construction
  line L446 (95.4538, 5.4429) -> (95.4538, 8.9706) construction
  line L447 (95.4538, 8.9706) -> (90.0364, 8.9706) construction
  line L448 (90.0364, 8.9706) -> (90.0364, 5.4429) construction
  line L449 (81.1468, 5.6558) -> (95.3079, 5.6558) construction
  line L450 (95.3079, 5.6558) -> (95.3079, 9.1836) construction
  line L451 (95.3079, 9.1836) -> (81.1468, 9.1836) construction
  line L452 (81.1468, 9.1836) -> (81.1468, 5.6558) construction
  line L453 (86.7207, 5.6558) -> (86.7224, 5.6558) construction
  line L454 (86.7224, 5.6558) -> (86.7224, 9.1836) construction
  line L455 (86.7224, 9.1836) -> (86.7207, 9.1836) construction
  line L456 (86.7207, 9.1836) -> (86.7207, 5.6558) construction
  line L457 (90.319, 5.6558) -> (95.7365, 5.6558) construction
  line L458 (95.7365, 5.6558) -> (95.7365, 9.1836) construction
  line L459 (95.7365, 9.1836) -> (90.319, 9.1836) construction
  line L460 (90.319, 9.1836) -> (90.319, 5.6558) construction
  line L461 (0.3101, -66.0432) -> (0.3101, -46.8075) construction
  line L462 (0.3101, -46.8075) -> (-3.2177, -46.8075) construction
  line L463 (-3.2177, -46.8075) -> (-3.2177, -66.0432) construction
  line L464 (-3.2177, -66.0432) -> (0.3101, -66.0432) construction
  line L465 (0.0265, -66.2554) -> (0.0265, -53.8186) construction
  line L466 (0.0265, -53.8186) -> (-3.5012, -53.8186) construction
  line L467 (-3.5012, -53.8186) -> (-3.5012, -66.2554) construction
  line L468 (-3.5012, -66.2554) -> (0.0265, -66.2554) construction
  line L469 (4.8596, -66.2554) -> (4.8596, -66.2537) construction
  line L470 (4.8596, -66.2537) -> (1.3318, -66.2537) construction
  line L471 (1.3318, -66.2537) -> (1.3318, -66.2554) construction
  line L472 (1.3318, -66.2554) -> (4.8596, -66.2554) construction
  line L473 (5.6357, -66.2554) -> (5.6357, -60.838) construction
  line L474 (5.6357, -60.838) -> (2.1079, -60.838) construction
  line L475 (2.1079, -60.838) -> (2.1079, -66.2554) construction
  line L476 (2.1079, -66.2554) -> (5.6357, -66.2554) construction
  line L477 (9.2428, -110.3136) -> (9.2428, -14.9931)
  line L478 (9.2428, -14.9931) -> (103.8578, -14.9931)
  line L479 (103.8578, -14.9931) -> (142.6281, 7.5847)
  line L480 (142.6281, 7.5847) -> (161.7839, -25.5411)
  line L481 (161.7839, -25.5411) -> (161.7839, -103.1522)
  line L482 (123.6486, -112.6772) -> (84.9842, -117.4397)
  line L483 (84.9842, -117.4397) -> (66.9572, -117.4397)
  line L484 (9.2428, -110.3136) -> (66.9572, -117.4397)
  line L485 (63.7469, -81.6328) -> (63.5469, -81.6328)
  line L486 (63.5469, -81.6328) -> (63.5469, -81.4328)
  line L487 (63.5469, -81.4328) -> (63.7469, -81.4328)
  line L488 (63.7469, -81.4328) -> (63.7469, -81.6328)
  line L489 (86.36, -81.6328) -> (86.56, -81.6328)
  line L490 (86.56, -81.6328) -> (86.56, -81.4328)
  line L491 (86.56, -81.4328) -> (86.36, -81.4328)
  line L492 (86.36, -81.4328) -> (86.36, -81.6328)
  line L493 (63.5469, -81.6328) -> (63.5469, -117.0186)
  line L494 (63.7469, -81.4328) -> (86.36, -81.4328)
  line L495 (86.56, -81.6328) -> (86.56, -117.2454)
  line L496 (63.5469, -81.4328) -> (57.5469, -81.4328)
  line L497 (57.5469, -81.4328) -> (57.5469, -87.4328)
  line L498 (86.56, -81.4328) -> (92.56, -81.4328)
  line L499 (9.2428, -51.1815) -> (27.2428, -51.1815)
  line L500 (161.7839, -48.2006) -> (143.7839, -48.2006)
  line L501 (57.5469, -81.4328) -> (27.2428, -81.4328)
  line L502 (27.2428, -81.4328) -> (27.2428, -51.1815)
  line L503 (143.7839, -48.2006) -> (143.7839, -81.4328)
  line L504 (143.7839, -81.4328) -> (92.56, -81.4328)
  line L505 (27.2428, -51.1815) -> (27.2428, -15.9328)
  line L506 (27.2428, -15.9328) -> (143.7839, -15.9328)
  line L507 (143.7839, -15.9328) -> (143.7839, -48.2006)
  line L508 (9.2428, -14.9931) -> (9.2428, 80.3275)
  line L509 (142.6281, 7.5847) -> (100.6075, 80.3275)
  line L510 (9.2428, 80.3275) -> (100.6075, 80.3275)
  line L511 (9.2428, 80.3275) -> (15.2428, 80.3275)
  line L512 (15.2428, 80.3275) -> (15.2428, 74.3275)
  line L513 (15.2428, 74.3275) -> (9.2428, 74.3275)
  line L514 (9.2428, 74.3275) -> (9.2428, 80.3275)
  line L515 (97.1443, 80.3275) -> (97.1443, 74.3275)
  line L516 (97.1443, 74.3275) -> (104.0735, 74.3275)
  circle A143 centre (97.1443, 74.3275) radius 6
  circle A144 centre (155.7839, -98.4665) radius 6
  circle A145 centre (15.2428, -105.0089) radius 6
  circle A146 centre (15.2428, 74.3275) radius 6
  circle A147 centre (155.7839, -27.151) radius 6
  line L517 (157.9757, -18.9558) -> (147.6976, -24.893)
  line L518 (161.7839, -33.151) -> (153.5462, -33.151)
  line L519 (161.7839, -92.4665) -> (149.7839, -92.4665)
  line L520 (149.7839, -92.4665) -> (149.7839, -106.1494)
  line L521 (9.2428, -99.0089) -> (21.2428, -99.0089)
  line L522 (21.2428, -99.0089) -> (21.2428, -111.7953)
  line L523 (91.1443, 80.3275) -> (91.1443, 68.3275)
  line L524 (91.1443, 68.3275) -> (107.5394, 68.3275)
  line L525 (9.2428, 68.3275) -> (21.2428, 68.3275)
  line L526 (21.2428, 68.3275) -> (21.2428, 80.3275)
  line L527 (27.2428, -81.4328) -> (21.2428, -81.4328)
  line L528 (21.2428, -81.4328) -> (21.2428, -75.4328)
  line L529 (27.2428, -15.9328) -> (21.2428, -15.9328)
  line L530 (21.2428, -15.9328) -> (21.2428, -21.9328)
  line L531 (143.7839, -15.9328) -> (143.7839, -9.9328)
  line L532 (143.7839, -9.9328) -> (119.7839, -9.9328)
  line L533 (143.7839, -81.4328) -> (86.56, -81.4328)
  line L534 (86.56, -81.4328) -> (86.56, -89.4328)
  line L535 (86.56, -89.4328) -> (143.7839, -89.4328)
  line L536 (143.7839, -89.4328) -> (143.7839, -81.4328)
  circle A148 centre (143.7839, -87.4328) radius 2
  circle A149 centre (88.56, -87.4328) radius 2
  circle A150 centre (141.7839, -15.9328) radius 2
  circle A151 centre (27.2428, -17.9328) radius 2
  circle A152 centre (29.2428, -81.4328) radius 2
  circle A153 centre (21.2428, -75.4328) radius 2.5
  circle A154 centre (21.2428, -21.9328) radius 2.5
  circle A155 centre (119.7839, -9.9328) radius 2.5
  circle A156 centre (57.5469, -87.4328) radius 2.5
  line L537 (92.56, -89.4328) -> (92.56, -95.4328)
  circle A157 centre (92.56, -95.4328) radius 2.5
  line L538 (143.7839, -89.4328) -> (149.7839, -89.4328)
  line L539 (149.7839, -89.4328) -> (149.7839, -83.4328)
  circle A158 centre (149.7839, -83.4328) radius 2.5
  line L540 (143.7839, -89.4328) -> (150.9524, -85.6429)
  line L541 (149.7839, -80.9328) -> (143.7839, -80.9328)
  line L542 (86.56, -89.4328) -> (90.3499, -96.6012)
  line L543 (92.56, -89.4328) -> (98.56, -89.4328)
  line L544 (98.56, -89.4328) -> (94.7701, -96.6012)
  line L545 (63.5469, -81.4328) -> (59.7571, -88.6012)
  line L546 (57.5469, -81.4328) -> (51.5469, -81.4328)
  line L547 (51.5469, -81.4328) -> (55.3368, -88.6012)
  line L548 (27.2428, -81.4328) -> (20.0743, -77.6429)
  line L549 (119.7839, -9.9328) -> (119.7839, -15.9328)
  line L550 (119.7839, -15.9328) -> (125.7839, -15.9328)
  line L551 (119.7839, -15.9328) -> (113.7839, -15.9328)
  line L552 (113.7839, -15.9328) -> (117.5738, -8.7643)
  line L553 (125.7839, -15.9328) -> (121.994, -8.7643)
  line L554 (27.2428, -15.9328) -> (20.0743, -19.7226)
  line L555 (21.2428, -21.9328) -> (27.2428, -21.9328)
  line L556 (27.2428, -21.9328) -> (27.2428, -27.9328)
  line L557 (27.2428, -27.9328) -> (20.0743, -24.1429)
  line L558 (21.2428, -75.4328) -> (27.2428, -75.4328)
  line L559 (27.2428, -75.4328) -> (27.2428, -69.4328)
  line L560 (27.2428, -69.4328) -> (20.0743, -73.2226)
  line L561 (18.8031, -81.7033) -> (9.2428, -81.7033)
  line L562 (142.7339, -107.9103) -> (142.7339, -30.6526)
  line L563 (161.7839, -25.5411) -> (155.7839, -27.151)
  line L564 (155.7839, -27.151) -> (142.7339, -30.6526)
  line L565 (146.7556, -76.7997) -> (142.7339, -76.7997)
  line L566 (146.7556, -76.7997) -> (150.7772, -76.7997)
  line L567 (150.7772, -76.7997) -> (150.7772, -74.7889)
  line L568 (150.7772, -76.7997) -> (150.7772, -78.8106)
  line L569 (142.7339, -82.8322) -> (150.7772, -78.8106)
  line L570 (150.7772, -74.7889) -> (142.7339, -70.7672)
  line L571 (142.7339, -76.7997) -> (142.7339, -70.7672)
  line L572 (142.7339, -107.9103) -> (123.6486, -112.6772)
  line L573 (123.6486, -112.6772) -> (118.0197, -90.1409)
  line L574 (161.7839, -103.1522) -> (145.5587, -103.1522)
  line L575 (126.1031, -100.5919) -> (140.1031, -100.5919)
  line L576 (140.1031, -100.5919) -> (140.1031, -86.5919)
  line L577 (140.1031, -86.5919) -> (126.1031, -86.5919)
  line L578 (126.1031, -86.5919) -> (126.1031, -100.5919)
  line L579 (140.1031, -100.5919) -> (140.1031, -103.2228)
  line L580 (121.9175, -105.7465) -> (132.0216, -103.2228)
  line L581 (132.0216, -103.2228) -> (140.1031, -103.2228)
  line L582 (140.1031, -103.2228) -> (142.7339, -103.2228)
  line L583 (125.5889, -108.1793) -> (124.8013, -105.0262)
  line L584 (146.7556, -37.8883) -> (150.7772, -37.8883)
  line L585 (150.7772, -37.8883) -> (150.7772, -40.3375)
  line L586 (143.7839, -37.8883) -> (143.7839, -43.9208)
  line L587 (146.7556, -37.8883) -> (143.7839, -37.8883)
  line L588 (150.7772, -37.8883) -> (150.7772, -28.4944)
  line L589 (144.7094, -55.4919) -> (144.7094, -48.4919)
  line L590 (144.7094, -48.4919) -> (157.6917, -48.4919)
  line L591 (157.6917, -48.4919) -> (161.7839, -46.6688)
  line L592 (161.7839, -46.6688) -> (161.7839, -42.1606)
  line L593 (150.7772, -40.3375) -> (157.6917, -40.3375)
  line L594 (157.6917, -40.3375) -> (161.7839, -42.1606)
  line L595 (157.6917, -44.4147) -> (157.6917, -48.4919)
  line L596 (157.6917, -44.4147) -> (157.6917, -40.3375)
  line L597 (143.7839, -43.9208) -> (142.7339, -43.9208)
  line L598 (142.7339, -43.9208) -> (150.7772, -40.3375)
  line L599 (144.7094, -48.4919) -> (142.7339, -48.4919)
  line L600 (157.6917, -48.4919) -> (161.7839, -48.4919)
  line L601 (157.6917, -40.3375) -> (161.7839, -40.3375)
  line L602 (146.7556, -76.7997) -> (146.7556, -80.8214)
  line L603 (146.7556, -76.7997) -> (146.7556, -72.7781)
  line L604 (146.7556, -72.7781) -> (142.7339, -72.7781)
  line L605 (146.7556, -72.7781) -> (150.7772, -72.7781)
  line L606 (150.7772, -72.7781) -> (150.7772, -74.7889)
  line L607 (150.7772, -78.8106) -> (150.7772, -80.8214)
  line L608 (150.7772, -80.8214) -> (146.7556, -80.8214)
  line L609 (142.7339, -80.8214) -> (146.7556, -80.8214)
  point P0 (66.3928, -86.8539)
  point P1 (66.3928, -89.3939)
  point P2 (66.3928, -91.9339)
  point P3 (66.3928, -94.4739)
  point P4 (66.3928, -97.0139)
  point P5 (66.3928, -99.5539)
  point P6 (66.3928, -102.0939)
  point P7 (66.3928, -104.6339)
  point P8 (66.3928, -107.1739)
  point P9 (66.3928, -109.7139)
  point P10 (66.3928, -112.2539)
  point P11 (85.4428, -108.8672)
  point P12 (85.4428, -106.3272)
  point P13 (84.5955, -104.6241)
  point P14 (85.4428, -101.2472)
  point P15 (85.4428, -98.7072)
  point P16 (85.4428, -96.1672)
  point P17 (85.4428, -93.6272)
  point P18 (85.4428, -91.0872)
  point P19 (85.4428, -88.5472)
  point P20 (85.4428, -86.0072)
  point P21 (85.4428, -83.4672)
  point P22 (84.4197, -112.2539)
  point P23 (84.4197, -109.7139)
  point P24 (84.4197, -107.1739)
  point P25 (84.4197, -104.6339)
  point P26 (84.4197, -102.0939)
  point P27 (84.4197, -99.5539)
  point P28 (84.4197, -97.0139)
  point P29 (84.4197, -94.4739)
  point P30 (84.4197, -91.9339)
  point P31 (84.4197, -89.3939)
  point P32 (84.4197, -86.8539)
  point P33 (84.4197, -84.3139)
  point P34 (69.1797, -84.3139)
  point P35 (69.1797, -86.8539)
  point P36 (69.1797, -89.3939)
  point P37 (69.1797, -91.9339)
  point P38 (69.1797, -94.4739)
  point P39 (69.1797, -97.0139)
  point P40 (69.1797, -99.5539)
  point P41 (69.1797, -102.0939)
  point P42 (69.1797, -104.6339)
  point P43 (69.1797, -107.1739)
  point P44 (69.1797, -109.7139)
  point P45 (69.1797, -112.2539)
  point P46 (81.8797, -89.3939)
  point P47 (79.3397, -89.3939)
  point P48 (76.7997, -89.3939)
  point P49 (162.1719, -101.6353)
  point P50 (162.1719, -100.8239)
  point P51 (162.1719, -100.0125)
  point P52 (148.3431, -37.8883)
  point P53 (116.84, -33.7256)
  point P54 (67.5217, -78.105)
  point P55 (20.3906, -34.0783)
  point P56 (132.4681, -10.2658)
  point P57 (125.1656, -102.5878)
  point P58 (159.2792, -44.4147)
  point P59 (72.1431, -18.8031)
  point P60 (96.3436, -34.2547)
  point P61 (148.3431, -76.7997)
  point P62 (29.9156, -91.2283)
  point P63 (156.3158, -33.8314)
  point P64 (156.3158, -36.3714)
  point P65 (85.4428, -103.7872)
  point P66 (151.2711, -21.9781)
  point P67 (141.7461, -5.4681)
  point P68 (116.9458, -19.7908)
  point P69 (86.1836, -29.3158)
  point P70 (59.5136, -29.3158)
  point P71 (40.4636, -24.5533)
  point P72 (21.4136, -24.5533)
  point P73 (134.7611, -31.5383)
  point P74 (116.6636, -45.9669)
  point P75 (97.6136, -48.3658)
  point P76 (78.5636, -50.7294)
  point P77 (59.5136, -48.3658)
  point P78 (40.4636, -43.6033)
  point P79 (21.4136, -43.6033)
  point P80 (135.7136, -55.4919)
  point P81 (116.6636, -65.0169)
  point P82 (97.6136, -67.4158)
  point P83 (78.5636, -69.7794)
  point P84 (59.5136, -67.4158)
  point P85 (40.4636, -62.6533)
  point P86 (21.4136, -62.6533)
  point P87 (135.7136, -74.5419)
  point P88 (116.6636, -84.0669)
  point P89 (97.6136, -86.4658)
  point P90 (78.5636, -88.8294)
  point P91 (59.5136, -86.4658)
  point P92 (40.4636, -81.7033)
  point P93 (21.4136, -81.7033)
  point P94 (135.7136, -93.5919)
  point P95 (116.6636, -103.1169)
  point P96 (97.6136, -105.5158)
  point P97 (78.5636, -107.8794)
  point P98 (59.5136, -105.5158)
  point P99 (40.4636, -100.7533)
  point P100 (21.4136, -100.7533)
  point P101 (156.3158, -66.5339)
  point P102 (156.3158, -69.0739)
  point P103 (160.1964, -57.9967)
  point P104 (160.1964, -52.9872)
  point P105 (145.6972, -55.4919)
  point P106 (145.6972, -52.9872)
  point P107 (160.1964, -96.0967)
  point P108 (160.1964, -91.0872)
  point P109 (145.6972, -93.5919)
  point P110 (145.6972, -91.0872)
  point P111 (105.3394, -83.82)
  point P112 (67.4158, -78.105)
  point P113 (116.7342, -33.7256)
  point P114 (96.2378, -34.2547)
  point P115 (72.0372, -18.8031)
  point P116 (29.845, -91.2283)
  point P117 (20.32, -34.0783)
  point P118 (132.4328, -10.2658)
  point P119 (148.2725, -76.7997)
  point P120 (159.2086, -44.4147)
  point P121 (148.2725, -37.8883)
  point P122 (125.095, -102.5878)
  dimension "d1" = 152.53
  dimension "d2" = 0.2
  dimension "d3" = 0.2
  dimension "d4" = 0.2
  dimension "d5" = 0.2
  dimension "d6" = 6
  dimension "d7" = 6
  dimension "d8" = 6
  dimension "d10" = 18
  dimension "d11" = 18
  dimension "d12" = 116.5411
  dimension "d13" = 65.5
  dimension "d14" = 0.9397
  dimension "d15" = 152.5411
  dimension "d16" = 95.3206
  dimension "d17" = 95.3206
  dimension "d18" = 6
  dimension "d19" = 6
  dimension "d20" = 6
  dimension "d22" = 12
  dimension "d23" = 12
  dimension "d24" = 12
  dimension "d25" = 12
  dimension "d26" = 12
  dimension "d27" = 6
  dimension "d28" = 6
  dimension "d29" = 6
  dimension "d30" = 6
  dimension "d31" = 6
  dimension "d32" = 24
  dimension "d33" = 8
  dimension "d34" = 4
  dimension "d35" = 4
  dimension "d36" = 4
  dimension "d37" = 4
  dimension "d38" = 4
  dimension "d39" = 5
  dimension "d40" = 5
  dimension "d41" = 5
  dimension "d42" = 5
  dimension "d43" = 6
  dimension "d44" = 6
  dimension "d45" = 5
  dimension "d46" = 6
  dimension "d47" = 6
  dimension "d48" = 5
  dimension "d49" = 6
  dimension "d50" = 6
  dimension "d51" = 6
  dimension "d52" = 6
  dimension "d53" = 6
  dimension "d54" = 6
  dimension "d55" = 9.5603
  dimension "d56" = 19.05
  dimension "d57" = 19.05
  dimension "d58" = 4.0217
  dimension "d59" = 4.0217
  dimension "d60" = 2.0108
  dimension "d61" = 2.0108
  dimension "d62" = 6.0325
  dimension "d63" = 6.0325
  dimension "d70" = 14.024
  dimension "d72" = 14
  dimension "d73" = 14
  dimension "d74" = 7
  dimension "d75" = 7
  dimension "d76" = 2.6308
  dimension "d77" = 2.6308
  dimension "d80" = 3.25
  dimension "d81" = 4.0217
  dimension "d82" = 4.0217
  dimension "d84" = 6.0325
  dimension "d87" = 7
  dimension "d88" = 65.987
  dimension "d89" = 65.987
  dimension "d90" = 65.987
  dimension "d91" = 4.0772
  dimension "d92" = 4.0772
  dimension "d93" = 4.0217
  dimension "d94" = 4.0217
  constraint coincident L0.start origin
  constraint horizontal L0
  constraint horizontal L485
  constraint vertical L486
  constraint horizontal L487
  constraint vertical L488
  constraint horizontal L489
  constraint vertical L490
  constraint horizontal L491
  constraint vertical L492
  constraint coincident L484 L493.end
  constraint perpendicular L485 L493
  constraint coincident L409 L495.end
  constraint perpendicular L9 L495
  constraint perpendicular L486 L496
  constraint perpendicular L496 L497
  constraint perpendicular L492 L498
  constraint coincident L477 L499.start
  constraint perpendicular L477 L499
  constraint coincident L481 L500.start
  constraint perpendicular L481 L500
  constraint perpendicular L497 L501
  constraint perpendicular L499 L502
  constraint perpendicular L503 L504